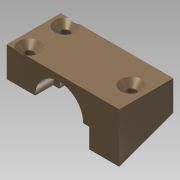
# Autodesk Inventor part: Lukker
Saved by Autodesk Inventor 2016 (Build 200138000, 138)
## iProperties
Created: 2015-07-28
Part Number: Lukker
Material: PLA Plastic
Document SubType Name: Modeling
Designer: Mathias L. Kjeldgaard
Density: 0.996477 g/cm^3
Appearance: Brindle
Author: Mathias L. Kjeldgaard
Autodesk Inventor part; units mm, degrees
ref_plane "YZ Plane" through (0, 0, 0) normal (1, 0, 0) x (0, 1, 0)
ref_plane "XZ Plane" through (0, 0, 0) normal (0, 1, 0) x (-1, 0, 0)
ref_plane "XY Plane" through (0, 0, 0) normal (0, 0, 1) x (1, 0, 0)
sketch "Sketch1" plane through (0, 0, 0) normal (0, 0, 1) x (1, 0, 0)
  line L0 (-13.216, 7.0679) -> (17.784, 7.0679) construction
  line L1 (17.784, 7.0679) -> (17.784, -7.9321) construction
  line L2 (17.784, -7.9321) -> (-13.216, -7.9321) construction
  line L3 (-13.216, -7.9321) -> (-13.216, 7.0679) construction
  circle A0 centre (-11.716, 5.5679) radius 1.5
  circle A1 centre (-11.716, -6.4321) radius 1.5
  circle A2 centre (16.284, -0.4321) radius 1.5
  line L4 (-16.216, 8.5679) -> (21.284, 8.5679)
  line L5 (21.284, 8.5679) -> (21.284, -9.4321)
  line L6 (21.284, -9.4321) -> (-16.216, -9.4321)
  line L7 (-16.216, -9.4321) -> (-16.216, 8.5679)
  point P0 (0, 0)
  dimension "d0" = 28
  dimension "d1" = 6
  dimension "d2" = 6
  dimension "d3" = 3
  dimension "d4" = 3
  dimension "d5" = 3
  dimension "d10" = 4.5
  dimension "d11" = 3
  dimension "d13" = 1.5
  dimension "d34" = 5
  constraints: 16 end point, 5 tangent, 4 parallel, 3 centre point, 2 horizontal, 2 perpendicular
  measures "d0" horizontal distance of A2.centre A1.centre
  measures "d1" vertical distance of A2.centre A1.centre
  measures "d2" vertical distance of A2.centre A0.centre
  measures "d3" diameter of A1
  measures "d4" diameter of A0
  measures "d5" diameter of A2
  measures "d10" distance from line of L7 A1.centre
  measures "d11" distance from line of L6 A1.centre
  measures "d13" distance between parallel lines of L4 L0
  measures "d34" distance from line of L5 A2.centre
extrude "Extrusion1" add sketch "Sketch1" along normal blind 10
sketch "Sketch3" plane through (-16.216, -9.4321, 10) normal (0, -1, 0) x (1, 0, 0)
  line L0 (37.5, -10) -> (0, -10) projected
  circle A0 centre (17.5, -10) radius 6 construction
  line L1 (23.5, -10) -> (23.5, -2.9049) construction
  circle A1 centre (17.5, -10) radius 8
  line L2 (0, -10) -> (0, 0) projected
  line L3 (9.5, -10) -> (9.5, -3.6397) construction
  point P0 (27.5, -10)
  point P1 (16.216, -10)
  dimension "d19" = 12
  dimension "d21" = 16
  dimension "d30" = 9.5
  constraints: 4 end point, 3 point on line, 2 horizontal alignment, 2 vertical, 1 coincident, 1 parallel, 1 perpendicular, 4 other
  measures "d30" distance between parallel lines of L3 L2
extrude "Extrusion3" cut sketch "Sketch3" against normal blind 6
sketch "Sketch4" plane through (-16.216, -3.4321, 10) normal (0, -1, 0) x (1, 0, 0)
  arc A0 (25.5, -10) -> (9.5, -10) centre (17.5, -10) ccw projected
  circle A1 centre (17.5, -10) radius 6
  point P0 (16.216, -10)
  dimension "d24" = 12
  constraints: 1 centre point, 1 coincident
  measures "d24" diameter of A1
extrude "Extrusion4" cut sketch "Sketch4" against normal blind 6
sketch "Sketch5" plane through (-16.216, 2.5679, 10) normal (0, -1, 0) x (1, 0, 0)
  arc A0 (23.5, -10) -> (11.5, -10) centre (17.5, -10) ccw projected
  circle A1 centre (17.5, -10) radius 8
  point P0 (16.216, -10)
  dimension "d27" = 16
  constraints: 1 centre point, 1 coincident
  measures "d27" diameter of A1
extrude "Extrusion5" cut sketch "Sketch5" against normal blind 19.5
sketch "Sketch6" plane through (21.284, -9.4321, 0) normal (1, 0, 0) x (0, 0, -1)
  line L0 (0, 18) -> (0, 0) projected
  line L1 (0, 18) -> (-10, 18) projected
  line L2 (0, 0) -> (-10, 0) projected
  line L3 (0, 18) -> (6.5515, 0)
  line L4 (0, 18) -> (12.9005, 18) construction
  line L5 (0, 0) -> (6.5515, 0)
  point P0 (0, 9.4321)
  dimension "d31" = 70
  constraints: 6 end point, 2 parallel
  measures "d31" angle of L4 L3
extrude "Extrusion6" add sketch "Sketch6" against normal blind 10
chamfer "Chamfer1" distance 2 angle 45 3 edges at (-13.216, 5.5679, 10) (-13.216, -6.4321, 10) (14.784, -0.4321, 10)
equation "\"d4\" = d3"
equation "\"d5\" = d3"
body "Solid1"
